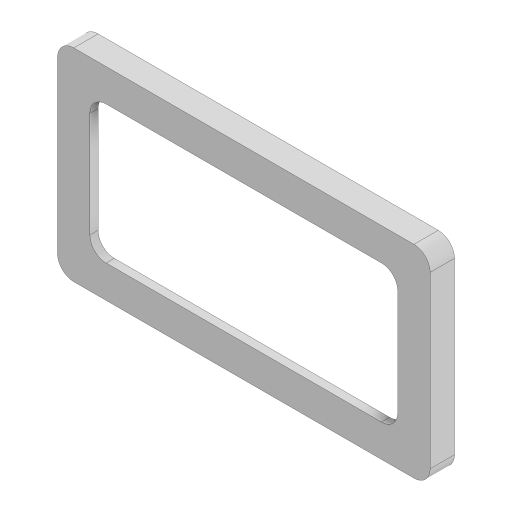
# Autodesk Inventor part: крышечка
Saved by Autodesk Inventor 2023.2 (Build 272271000, 271)
## iProperties
Created: 2023-11-25
Part Number: крышечка
Material: Типовые
Document SubType Name: Modeling
Designer: matvey
Density: 1 g/cm^3
Appearance: По умолчанию
Author: matvey
Autodesk Inventor part; units mm, degrees
ref_plane "YZ Plane" through (0, 0, 0) normal (1, 0, 0) x (0, 1, 0)
ref_plane "XZ Plane" through (0, 0, 0) normal (0, 1, 0) x (-1, 0, 0)
ref_plane "XY Plane" through (0, 0, 0) normal (0, 0, 1) x (1, 0, 0)
sketch "Эскиз1" plane through (0, 0, 0) normal (0, 0, 1) x (1, 0, 0)
  line L0 (19, -8.5) -> (-19, -8.5)
  line L1 (-19, -8.5) -> (-19, 8.5)
  line L2 (-19, 8.5) -> (19, 8.5)
  line L3 (19, 8.5) -> (19, -8.5)
  line L4 (19, -8.5) -> (-19, 8.5) construction
  line L5 (-19, -8.5) -> (19, 8.5) construction
  line L6 (22, -11.5) -> (-22, -11.5)
  line L7 (-22, -11.5) -> (-22, 11.5)
  line L8 (-22, 11.5) -> (22, 11.5)
  line L9 (22, 11.5) -> (22, -11.5)
  line L10 (22, -11.5) -> (-22, 11.5) construction
  line L11 (-22, -11.5) -> (22, 11.5) construction
  point P0 (0, 0)
  dimension "d0" = 44
  dimension "d1" = 23
  dimension "d2" = 3
  dimension "d3" = 3
  constraints: 24 end point, 4 midpoint, 4 parallel, 2 horizontal, 2 perpendicular
  measures "d0" distance between parallel lines of L9 L7
  measures "d1" distance between parallel lines of L6 L8
  measures "d2" distance between parallel lines of L2 L8
  measures "d3" distance between parallel lines of L9 L3
extrude "Выдавливание1" add sketch "Эскиз1" along normal blind 1
sketch "Эскиз2" plane through (0, 0, 1) normal (0, 0, 1) x (1, 0, 0)
  line L0 (22, 11.5) -> (-22, 11.5) projected
  line L1 (-22, 11.5) -> (-22, -11.5) projected
  line L2 (-22, -11.5) -> (22, -11.5) projected
  line L3 (22, -11.5) -> (22, 11.5) projected
  line L4 (19, -8.5) -> (-19, -8.5) projected
  line L5 (-19, -8.5) -> (-19, 8.5) projected
  line L6 (-19, 8.5) -> (19, 8.5) projected
  line L7 (19, 8.5) -> (19, -8.5) projected
  line L8 (-23, 12.5) -> (23, 12.5)
  line L9 (23, 12.5) -> (23, -12.5)
  line L10 (23, -12.5) -> (-23, -12.5)
  line L11 (-23, -12.5) -> (-23, 12.5)
  point P0 (0, 0)
  dimension "d6" = 1
  constraints: 8 end point, 3 other
  measures "d6" distance between parallel lines of L0 L8
extrude "Выдавливание2" add sketch "Эскиз2" against normal blind 3 contours L8 L9 L10 L11
fillet "Сопряжение1" radius 2 8 edges at (23, 12.5, -0.5) (-23, 12.5, -0.5) (-23, -12.5, -0.5) (23, -12.5, -0.5) (-19, 8.5, 0.5) (19, 8.5, 0.5) (19, -8.5, 0.5) (-19, -8.5, 0.5)
